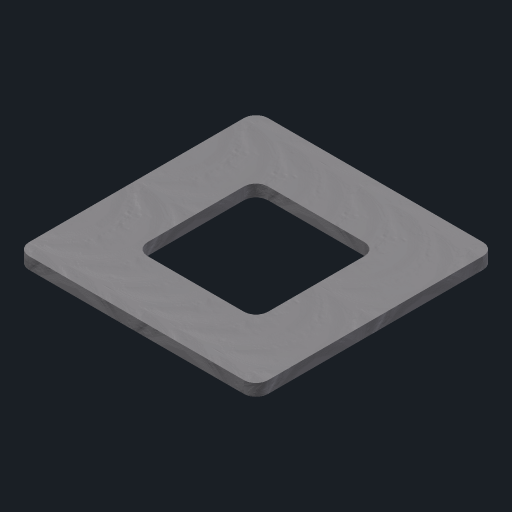
# Autodesk Inventor part: PATA
Saved by Autodesk Inventor 2024.3 (Build 283343000, 343)
## iProperties
Created: 2024-08-10
Part Number: PATA
Material: Steel, Mild, Welded
Document SubType Name: Modeling
Designer: Niler
Density: 7.85 g/cm^3
Appearance: Weld - Steel Mild
Author: Niler
Autodesk Inventor part; units mm, degrees
ref_plane "YZ Plane" through (0, 0, 0) normal (1, 0, 0) x (0, 1, 0)
ref_plane "XZ Plane" through (0, 0, 0) normal (0, 1, 0) x (-1, 0, 0)
ref_plane "XY Plane" through (0, 0, 0) normal (0, 0, 1) x (1, 0, 0)
sketch "Sketch1" plane through (0, 0, 0) normal (0, 1, 0) x (-1, 0, 0)
  line L0 (-25.2, 25.2) -> (25.2, 25.2)
  line L1 (25.2, 25.2) -> (25.2, -25.2)
  line L2 (25.2, -25.2) -> (-25.2, -25.2)
  line L3 (-25.2, -25.2) -> (-25.2, 25.2)
  line L4 (-25.2, 25.2) -> (25.2, -25.2) construction
  line L5 (25.2, 25.2) -> (-25.2, -25.2) construction
  line L6 (-50, 50) -> (50, 50)
  line L7 (50, 50) -> (50, -50)
  line L8 (50, -50) -> (-50, -50)
  line L9 (-50, -50) -> (-50, 50)
  line L10 (-50, 50) -> (50, -50) construction
  line L11 (50, 50) -> (-50, -50) construction
  point P0 (0, 0)
  dimension "d0" = 50.4
  dimension "d1" = 100
  constraints: 24 end point, 4 midpoint, 4 parallel, 4 perpendicular, 2 horizontal
  measures "d0" distance of L0.end L1.end
  measures "d1" distance of L6.end L7.end
extrude "Extrusion1" add sketch "Sketch1" along normal blind 5
fillet "Fillet1" radius 5 8 edges at (50, 2.5, 50) (50, 2.5, -50) (-50, 2.5, 50) (-50, 2.5, -50) (-25.2, 2.5, -25.2) (25.2, 2.5, -25.2) (-25.2, 2.5, 25.2) (25.2, 2.5, 25.2)
body "Solid1"
